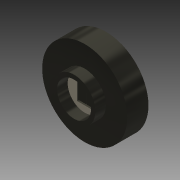
# Autodesk Inventor part: Lens
Saved by Autodesk Inventor 2015 SP1 (Build 190203100, 203)
## iProperties
Created: 2015-05-04
Part Number: Lens
Material: Generic
Document SubType Name: Modeling
Designer: Brandon
Density: 1 g/cm^3
Appearance: Gunmetal
Author: Brandon
Autodesk Inventor part; units mm, degrees
ref_plane "YZ Plane" through (0, 0, 0) normal (1, 0, 0) x (0, 1, 0)
ref_plane "XZ Plane" through (0, 0, 0) normal (0, 1, 0) x (-1, 0, 0)
ref_plane "XY Plane" through (0, 0, 0) normal (0, 0, 1) x (1, 0, 0)
sketch "Sketch1" plane through (0, 0, 0) normal (0, 0, 1) x (1, 0, 0)
  line L0 (-37.1, -32.05) -> (37.1, -32.05) projected
  line L1 (37.1, 32.05) -> (-37.1, 32.05) projected
  circle A0 centre (0, 0) radius 25.4
  line L2 (37.1, -32.05) -> (37.1, 32.05) projected
  line L3 (-37.1, 32.05) -> (-37.1, -32.05) projected
  dimension "d0" = 50.8
  constraints: 1 centre point, 1 coincident
  measures "d0" diameter of A0
extrude "Lens body" add sketch "Sketch1" along normal blind 12.7 contours A0
sketch "Sketch2" plane through (0, 0, 12.7) normal (0, 0, 1) x (1, 0, 0)
  circle A0 centre (0, 0) radius 25.4 projected
  circle A1 centre (0, 0) radius 12.7
  dimension "d3" = 25.4
  constraints: 1 centre point, 1 coincident
  measures "d3" diameter of A1
extrude "Ring" add sketch "Sketch2" along normal blind 6.35 contours A1
sketch "Sketch5" plane through (0, 0, 19.05) normal (0, 0, 1) x (1, 0, 0)
  circle A0 centre (0, 0) radius 12.7 projected
  circle A1 centre (0, 0) radius 10.16
  dimension "d14" = 2.54
  constraints: 1 centre point
  measures "d14" radial gap between concentric circles of A0 A1
extrude "Pit" cut sketch "Sketch5" against normal blind 6.35 contours A1
sketch "Sketch6" plane through (0, 0, 12.7) normal (0, 0, 1) x (1, 0, 0)
  line L0 (4.445, 6.35) -> (-4.445, 6.35)
  line L1 (-4.445, 6.35) -> (-4.445, -6.35)
  line L2 (-4.445, -6.35) -> (4.445, -6.35)
  line L3 (4.445, -6.35) -> (4.445, 6.35)
  line L4 (4.445, 6.35) -> (-4.445, -6.35) construction
  line L5 (-4.445, 6.35) -> (4.445, -6.35) construction
  point P0 (0, 0)
  dimension "d17" = 12.7
  dimension "d18" = 8.89
  constraints: 12 end point, 2 midpoint, 2 parallel, 1 horizontal, 1 perpendicular
  measures "d17" distance of L0.end L1.end
  measures "d18" distance of L1.end L2.end
extrude "Shutters" cut sketch "Sketch6" against normal blind 1
sketch "Sketch7" plane through (0, 0, 11.7) normal (0, 0, 1) x (1, 0, 0)
  line L0 (-4.445, 6.35) -> (4.445, 6.35) projected
  line L1 (-4.445, -6.35) -> (-4.445, 6.35) projected
  line L2 (4.445, -6.35) -> (-4.445, -6.35) projected
  line L3 (4.445, 6.35) -> (4.445, -6.35) projected
  line L4 (4.445, -6.35) -> (-4.445, -6.35) projected
  line L5 (-0.25, 6.35) -> (0.25, 6.35)
  line L6 (0.25, 6.35) -> (0.25, -6.35)
  line L7 (0.25, -6.35) -> (-0.25, -6.35)
  line L8 (-0.25, -6.35) -> (-0.25, 6.35)
  line L9 (-0.25, 6.35) -> (0.25, -6.35) construction
  line L10 (0.25, 6.35) -> (-0.25, -6.35) construction
  point P0 (0, 0)
  dimension "d21" = 0.5
  constraints: 12 end point, 2 midpoint, 2 parallel, 1 horizontal, 1 perpendicular, 1 point on line
  measures "d21" distance of L6.end L7.end
extrude "Extrusion7" cut sketch "Sketch7" against normal blind 0.5 contours L0 L6 L2 L8
body "Solid1"
